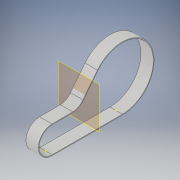
# Autodesk Inventor part: paseknowy
Saved by Autodesk Inventor 2019 (Build 230136000, 136)
## iProperties
Created: 2020-05-17
Part Number: paseknowy
Material: Generic
Document SubType Name: Modeling
Designer: estee
Density: 1 g/cm^3
Appearance: Default
Author: estee
Autodesk Inventor part; units mm, degrees
ref_plane "YZ Plane" through (0, 0, 0) normal (1, 0, 0) x (0, 1, 0)
ref_plane "XZ Plane" through (0, 0, 0) normal (0, 1, 0) x (-1, 0, 0)
ref_plane "Work Plane1" through (0, 0, 18) normal (0, 0, 1) x (1, 0, 0)
sketch "Sketch1" plane through (0, 0, 0) normal (1, 0, 0) x (0, 1, 0)
  arc A0 (-3.5373, 37.5621) -> (-14.976, 34) centre (-8.702, 34) ccw
  line L0 (0, 54.2276) -> (0, -32.966) construction
  line L1 (0, -32.966) -> (0, 54.2276) projected
  line L2 (-24.1835, 0) -> (27.9587, 0) construction
  line L3 (-14.976, 0) -> (-14.976, 34)
  line L4 (-24.1835, 18) -> (27.9587, 18) construction
  arc A1 (-2.428, 34) -> (-14.976, 34) centre (-8.702, 34) ccw
  arc A2 (-2.335, 24) -> (0.4081, 18.7817) centre (4, 24) ccw
  line L5 (-0.319, 19.362) -> (-0.4473, 19.4885)
  line L6 (-2.335, 24) -> (-2.428, 34)
  line L7 (9.2809, 11.7535) -> (0.4081, 18.7817)
  arc A3 (-14.976, 0) -> (9.2809, 11.7535) centre (0, 0) ccw
  line L8 (9.5142, 12.0484) -> (0.6316, 19.0844)
  arc A4 (-1.959, 24.0017) -> (0.6316, 19.0844) centre (4, 24) ccw
  line L9 (-1.959, 24.0017) -> (-2.052, 34.0018)
  arc A5 (-2.052, 34.0018) -> (-15.352, 34) centre (-8.702, 34) ccw
  line L10 (-15.352, 34) -> (-15.352, 0)
  arc A6 (-15.352, 0) -> (9.5142, 12.0484) centre (0, 0) ccw
  dimension "d2" = 12.548
  dimension "d3" = 34
  dimension "d4" = 8.702
  dimension "d8" = 12.67
  dimension "d9" = 4
  dimension "d10" = 6
  dimension "d11" = 29.952
  dimension "d12" = 0.376
  constraints: 15 point on circle, 14 end point, 7 centre point, 2 tangent, 1 coincident, 1 concentric, 1 point on line, 6 other
  measures "d2" diameter of A0
  measures "d3" vertical distance of point (0, 0) A0.centre
  measures "d4" distance from line of L0 A0.centre
  measures "d8" diameter of A2
  measures "d9" distance from line of L0 A2.centre
  measures "d11" diameter of A3
  measures "d12" radial gap between concentric circles of A3 A6
extrude "Extrusion1" add sketch "Sketch1" along normal mid plane 6 contours A0 L3 A3 L1 A6 L10 A5 L9 A4 A2 L6 A1 | A3 L7 A2 L1 A4 L8 A6
equation "\"start\" = d3"
equation "\"d7\" = start"
body "Solid1"
